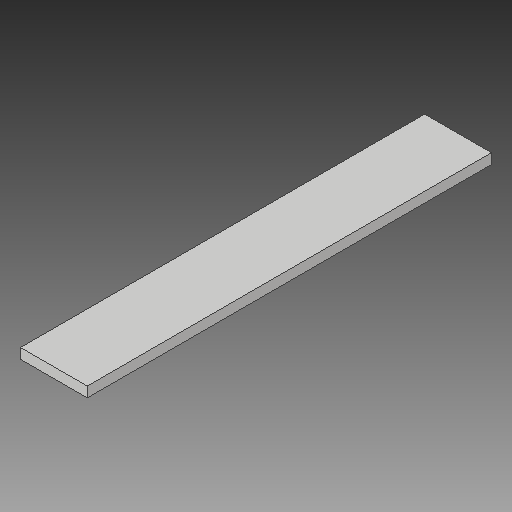
# Autodesk Inventor part: core_lightStrip_R
Saved by Autodesk Inventor 2017 (Build 210142000, 142)
## iProperties
Created: 2017-05-29
Part Number: core_lightStrip_R
Material: Generic
Document SubType Name: Modeling
Designer: Paolo
Density: 1 g/cm^3
Appearance: Default
Mass: 6.97368 g
Surface Area: 54.7832 cm^2
Volume: 6.97368 cm^3
Author: Paolo
Autodesk Inventor part; units mm, degrees
ref_plane "YZ Plane" through (0, 0, 0) normal (1, 0, 0) x (0, 1, 0)
ref_plane "XZ Plane" through (0, 0, 0) normal (0, 1, 0) x (-1, 0, 0)
ref_plane "XY Plane" through (0, 0, 0) normal (0, 0, 1) x (1, 0, 0)
sketch "Sketch1" plane through (0, 0, 0) normal (0, 1, 0) x (-1, 0, 0)
  line L0 (-9.8, 59.3) -> (9.8, 59.3)
  line L1 (9.8, 59.3) -> (9.8, -59.3)
  line L2 (9.8, -59.3) -> (-9.8, -59.3)
  line L3 (-9.8, -59.3) -> (-9.8, 59.3)
  line L4 (-9.8, 59.3) -> (9.8, -59.3) construction
  line L5 (9.8, 59.3) -> (-9.8, -59.3) construction
  point P0 (0, 0)
  dimension "d0" = 19.6
  dimension "d1" = 118.6
  constraints: 12 end point, 2 midpoint, 2 parallel, 1 horizontal, 1 perpendicular
  measures "d0" distance of L1.end L2.end
  measures "d1" distance of L0.end L1.end
extrude "Extrusion1" add sketch "Sketch1" along normal blind 3
body "Solid1"
